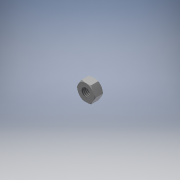
# Autodesk Inventor part: 24-706-8
Saved by Autodesk Inventor 2018 (Build 220105000, 105)
## iProperties
Created: 2004-11-18
Part Number: 24-706-8
Material: Stainless Steel, Austenitic
Document SubType Name: Modeling
Designer: Autodesk, Inc.
Manufacturer: Standard
Standards Organization: Custom
Description: Hexagon Nut, M8
Catalog Web Link: http://www.parker.com/ead/cm1.asp?cmid=809
Vendor: PARKER IPS
Mass: 6.05208 g
Surface Area: 6.5618 cm^2
Volume: 0.753683 cm^3
Density: 8.03 g/cm^3
Appearance: Steel
CAGE: 1LJX3
Dept. ID: Product Design
Description #2: ---
Finish #1: ---
Finish #2: ---
Material ID: ---
Project Number: ---
Author: Autodesk, Inc.
Autodesk Inventor part; units mm, degrees
ref_plane "YZ Plane" through (0, 0, 0) normal (1, 0, 0) x (0, 1, 0)
ref_plane "XZ Plane" through (0, 0, 0) normal (0, 1, 0) x (-1, 0, 0)
ref_plane "XY Plane" through (0, 0, 0) normal (0, 0, 1) x (1, 0, 0)
sketch "Sketch1" plane through (0, 0, 0) normal (0, 0, 1) x (1, 0, 0)
  line L0 (3.7528, -6.5) -> (-3.7528, -6.5)
  line L1 (-3.7528, -6.5) -> (-7.5056, 0)
  line L2 (-7.5056, 0) -> (-3.7528, 6.5)
  line L3 (-3.7528, 6.5) -> (3.7528, 6.5)
  line L4 (3.7528, 6.5) -> (7.5056, 0)
  line L5 (7.5056, 0) -> (3.7528, -6.5)
  point P0 (0, 0)
  dimension "Width" = 13
  constraints: 12 end point, 1 horizontal, 12 other
  measures "Width" distance between parallel lines of L0 L3
extrude "Extrusion1" add sketch "Sketch1" along normal mid plane 6.8
sketch "Sketch2" plane through (0, 0, 0) normal (0, 1, 0) x (-1, 0, 0)
  line L0 (-7.5056, 3.4) -> (-7.5056, -3.4) projected
  line L1 (-3.7528, -3.4) -> (-7.5056, -3.4) projected
  line L2 (-7.5056, -2.72) -> (-6.5, -3.4)
  line L3 (1.5011, 0) -> (-9.0067, 0) construction
  line L4 (0, -4.76) -> (0, 4.76) construction
  point P0 (0, 0)
  dimension "d3" = 13
  dimension "d4" = 5.44
  constraints: 2 end point, 2 point on line
  measures "d3" diameter of L2.end L4
  measures "d4" diameter of L2.start L3
revolve "Revolution1" cut sketch "Sketch2" angle 360 about axis through (0, 0, -10) along (0, 0, 1)
mirror "Mirror1" about plane through (0, 0, 0) normal (0, 0, 1) of "Revolution1"
sketch "Sketch3" plane through (0, 0, -3.4) normal (0, 0, -1) x (-1, 0, 0)
  point P0 (0, 0)
hole "Hole1" at (0, 0, -3.4) direction (0, 0, 1) diameter 6.647 end through all thread size "M8x1.25" class "6H" standard "ANSI Metric M Profile"
equation "\"d3\" = Width"
equation "\"d4\" = 0.8 * Height"
equation "\"Height\" = 6.8"
body "Solid1"
